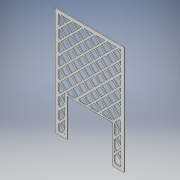
# Autodesk Inventor part: 2AM-17-07-Belly Pan
Saved by Autodesk Inventor 2017 (Build 210142000, 142)
## iProperties
Created: 2017-12-28
Part Number: 2AM-17-07-Belly Pan
Material: Generic
Document SubType Name: Modeling
Designer: anikasoojin
Density: 1 g/cm^3
Appearance: Default
Author: anikasoojin
Autodesk Inventor part; units mm, degrees
ref_plane "YZ Plane" through (0, 0, 0) normal (1, 0, 0) x (0, 1, 0)
ref_plane "XZ Plane" through (0, 0, 0) normal (0, 1, 0) x (-1, 0, 0)
ref_plane "XY Plane" through (0, 0, 0) normal (0, 0, 1) x (1, 0, 0)
sketch "Sketch1" plane through (0, 0, 0) normal (0, 0, 1) x (1, 0, 0)
  line L0 (80.4678, 8.0008) -> (613.8678, 8.0008)
  line L1 (613.8678, 8.0008) -> (613.8678, -830.1992)
  line L2 (80.4678, -830.1992) -> (80.4678, 8.0008)
  line L3 (572.8411, -17.3992) -> (588.4678, -33.0259)
  line L4 (563.8608, -26.3795) -> (588.4678, -50.9864)
  line L5 (588.4678, -17.3992) -> (572.8411, -17.3992)
  line L6 (588.4678, -33.0259) -> (588.4678, -17.3992)
  line L7 (483.0385, -17.3992) -> (518.9595, -53.3203)
  line L8 (554.8806, -17.3992) -> (518.9595, -53.3203)
  line L9 (474.0583, -26.3795) -> (509.9793, -62.3005)
  line L10 (563.8608, -26.3795) -> (527.9398, -62.3005)
  line L11 (588.4678, -76.6506) -> (588.4678, -50.9864)
  line L12 (565.3788, -99.7395) -> (588.4678, -76.6506)
  line L13 (527.9398, -62.3005) -> (565.3788, -99.7395)
  line L14 (574.3591, -108.7198) -> (588.4678, -122.8285)
  line L15 (518.9595, -71.2808) -> (556.3985, -108.7198)
  line L16 (565.3788, -117.7) -> (588.4678, -140.789)
  line L17 (574.3591, -108.7198) -> (588.4678, -94.6111)
  line L18 (588.4678, -122.8285) -> (588.4678, -94.6111)
  line L19 (554.8806, -17.3992) -> (483.0385, -17.3992)
  line L20 (465.078, -17.3992) -> (429.157, -53.3203)
  line L21 (393.236, -17.3992) -> (429.157, -53.3203)
  line L22 (384.2557, -26.3795) -> (420.1767, -62.3005)
  line L23 (474.0583, -26.3795) -> (438.1372, -62.3005)
  line L24 (438.1372, -62.3005) -> (474.0583, -98.2215)
  line L25 (509.9793, -62.3005) -> (474.0583, -98.2215)
  line L26 (429.157, -71.2808) -> (465.078, -107.2018)
  line L27 (518.9595, -71.2808) -> (483.0385, -107.2018)
  line L28 (520.4775, -144.6408) -> (556.3985, -108.7198)
  line L29 (483.0385, -107.2018) -> (520.4775, -144.6408)
  line L30 (474.0583, -116.1821) -> (511.4973, -153.6211)
  line L31 (529.4578, -153.6211) -> (565.3788, -117.7)
  line L32 (565.7758, -189.9391) -> (588.4678, -167.2472)
  line L33 (529.4578, -153.6211) -> (565.7758, -189.9391)
  line L34 (576.6156, -200.7789) -> (588.4678, -212.631)
  line L35 (520.4775, -162.6013) -> (556.7956, -198.9194)
  line L36 (567.6353, -209.7591) -> (588.4678, -230.5916)
  line L37 (576.6156, -200.7789) -> (588.4678, -188.9267)
  line L38 (588.4678, -167.2472) -> (588.4678, -140.789)
  line L39 (465.078, -107.2018) -> (429.157, -143.1228)
  line L40 (474.0583, -116.1821) -> (438.1372, -152.1031)
  line L41 (438.1372, -152.1031) -> (475.5762, -189.5421)
  line L42 (475.5762, -189.5421) -> (511.4973, -153.6211)
  line L43 (429.157, -161.0833) -> (466.596, -198.5223)
  line L44 (484.5565, -198.5223) -> (520.4775, -162.6013)
  line L45 (465.078, -17.3992) -> (393.236, -17.3992)
  line L46 (303.4334, -17.3992) -> (339.3544, -53.3203)
  line L47 (375.2754, -17.3992) -> (339.3544, -53.3203)
  line L48 (294.4531, -26.3795) -> (330.3742, -62.3005)
  line L49 (384.2557, -26.3795) -> (348.3347, -62.3005)
  line L50 (348.3347, -62.3005) -> (384.2557, -98.2215)
  line L51 (393.236, -107.2018) -> (429.157, -143.1228)
  line L52 (420.1767, -62.3005) -> (384.2557, -98.2215)
  line L53 (339.3544, -71.2808) -> (375.2754, -107.2018)
  line L54 (384.2557, -116.1821) -> (420.1767, -152.1031)
  line L55 (429.157, -71.2808) -> (393.236, -107.2018)
  line L56 (375.2754, -107.2018) -> (339.3544, -143.1228)
  line L57 (384.2557, -116.1821) -> (348.3347, -152.1031)
  line L58 (303.4334, -107.2018) -> (339.3544, -143.1228)
  line L59 (330.3742, -62.3005) -> (294.4531, -98.2215)
  line L60 (294.4531, -116.1821) -> (330.3742, -152.1031)
  line L61 (339.3544, -71.2808) -> (303.4334, -107.2018)
  line L62 (375.2754, -17.3992) -> (303.4334, -17.3992)
  line L63 (285.4729, -17.3992) -> (213.6308, -17.3992)
  line L64 (195.6703, -17.3992) -> (123.8283, -17.3992)
  line L65 (213.6308, -17.3992) -> (249.5519, -53.3203)
  line L66 (258.5321, -62.3005) -> (294.4531, -98.2215)
  line L67 (285.4729, -17.3992) -> (249.5519, -53.3203)
  line L68 (204.6506, -26.3795) -> (240.5716, -62.3005)
  line L69 (249.5519, -71.2808) -> (285.4729, -107.2018)
  line L70 (294.4531, -26.3795) -> (258.5321, -62.3005)
  line L71 (123.8283, -17.3992) -> (159.7493, -53.3203)
  line L72 (204.6506, -26.3795) -> (168.7296, -62.3005)
  line L73 (168.7296, -62.3005) -> (204.6506, -98.2215)
  line L74 (240.5716, -62.3005) -> (204.6506, -98.2215)
  line L75 (249.5519, -71.2808) -> (213.6308, -107.2018)
  line L76 (285.4729, -107.2018) -> (249.5519, -143.1228)
  line L77 (213.6308, -107.2018) -> (249.5519, -143.1228)
  line L78 (204.6506, -116.1821) -> (240.5716, -152.1031)
  line L79 (294.4531, -116.1821) -> (258.5321, -152.1031)
  line L80 (330.3742, -152.1031) -> (294.4531, -188.0241)
  line L81 (258.5321, -152.1031) -> (294.4531, -188.0241)
  line L82 (249.5519, -161.0833) -> (285.4729, -197.0044)
  line L83 (339.3544, -161.0833) -> (303.4334, -197.0044)
  line L84 (303.4334, -197.0044) -> (339.3544, -232.9254)
  line L85 (339.3544, -161.0833) -> (375.2754, -197.0044)
  line L86 (420.1767, -152.1031) -> (384.2557, -188.0241)
  line L87 (375.2754, -197.0044) -> (339.3544, -232.9254)
  line L88 (348.3347, -152.1031) -> (384.2557, -188.0241)
  line L89 (195.6703, -17.3992) -> (159.7493, -53.3203)
  line L90 (150.769, -62.3005) -> (114.848, -98.2215)
  line L91 (105.8678, -17.3992) -> (150.769, -62.3005)
  line L92 (159.7493, -71.2808) -> (195.6703, -107.2018)
  line L93 (105.8678, -89.2413) -> (114.848, -98.2215)
  line L94 (159.7493, -71.2808) -> (123.8283, -107.2018)
  line L95 (114.848, -116.1821) -> (105.8678, -125.1623)
  line L96 (105.8678, -17.3992) -> (105.8678, -89.2413)
  line L97 (114.848, -116.1821) -> (150.769, -152.1031)
  line L98 (195.6703, -107.2018) -> (159.7493, -143.1228)
  line L99 (150.769, -152.1031) -> (115.9232, -186.9489)
  line L100 (123.8283, -107.2018) -> (159.7493, -143.1228)
  line L101 (204.6506, -116.1821) -> (168.7296, -152.1031)
  line L102 (240.5716, -152.1031) -> (204.6506, -188.0241)
  line L103 (168.7296, -152.1031) -> (204.6506, -188.0241)
  line L104 (159.7493, -161.0833) -> (195.6703, -197.0044)
  line L105 (249.5519, -161.0833) -> (213.6308, -197.0044)
  line L106 (105.8678, -176.8934) -> (115.9232, -186.9489)
  line L107 (159.7493, -161.0833) -> (124.9035, -195.9292)
  line L108 (114.848, -205.9846) -> (105.8678, -214.9649)
  line L109 (588.4678, -212.631) -> (588.4678, -188.9267)
  line L110 (588.4678, -257.8438) -> (588.4678, -230.5916)
  line L111 (575.1531, -289.1189) -> (588.4678, -302.4336)
  line L112 (566.1728, -298.0992) -> (588.4678, -320.3941)
  line L113 (566.1728, -280.1387) -> (588.4678, -257.8438)
  line L114 (575.1531, -289.1189) -> (588.4678, -275.8043)
  line L115 (475.5762, -207.5026) -> (511.8943, -243.8206)
  line L116 (522.734, -254.6604) -> (557.1926, -289.1189)
  line L117 (520.8745, -234.8404) -> (556.7956, -198.9194)
  line L118 (484.5565, -198.5223) -> (520.8745, -234.8404)
  line L119 (531.7143, -245.6801) -> (566.1728, -280.1387)
  line L120 (531.7143, -245.6801) -> (567.6353, -209.7591)
  line L121 (393.236, -197.0044) -> (430.675, -234.4434)
  line L122 (430.675, -234.4434) -> (466.596, -198.5223)
  line L123 (384.2557, -205.9846) -> (421.6947, -243.4236)
  line L124 (439.6552, -243.4236) -> (475.5762, -207.5026)
  line L125 (429.157, -161.0833) -> (393.236, -197.0044)
  line L126 (384.2557, -205.9846) -> (348.3347, -241.9056)
  line L127 (294.4531, -205.9846) -> (330.3742, -241.9056)
  line L128 (475.9733, -279.7417) -> (511.8943, -243.8206)
  line L129 (439.6552, -243.4236) -> (475.9733, -279.7417)
  line L130 (430.675, -252.4039) -> (466.993, -288.7219)
  line L131 (486.813, -290.5814) -> (522.734, -254.6604)
  line L132 (105.8678, -125.1623) -> (105.8678, -176.8934)
  line L133 (195.6703, -197.0044) -> (160.8245, -231.8502)
  line L134 (150.769, -241.9056) -> (114.848, -277.8267)
  line L135 (124.9035, -195.9292) -> (160.8245, -231.8502)
  line L136 (114.848, -205.9846) -> (150.769, -241.9056)
  line L137 (204.6506, -205.9846) -> (169.8048, -240.8304)
  line L138 (285.4729, -197.0044) -> (249.5519, -232.9254)
  line L139 (213.6308, -197.0044) -> (249.5519, -232.9254)
  line L140 (294.4531, -205.9846) -> (258.5321, -241.9056)
  line L141 (204.6506, -205.9846) -> (240.5716, -241.9056)
  line L142 (258.5321, -241.9056) -> (294.4531, -277.8267)
  line L143 (330.3742, -241.9056) -> (294.4531, -277.8267)
  line L144 (249.5519, -250.8859) -> (285.4729, -286.8069)
  line L145 (339.3544, -250.8859) -> (303.4334, -286.8069)
  line L146 (339.3544, -250.8859) -> (376.7934, -288.3249)
  line L147 (385.7737, -279.3446) -> (421.6947, -243.4236)
  line L148 (348.3347, -241.9056) -> (385.7737, -279.3446)
  line L149 (394.7539, -288.3249) -> (430.675, -252.4039)
  line L150 (394.7539, -288.3249) -> (431.072, -324.643)
  line L151 (431.072, -324.643) -> (466.993, -288.7219)
  line L152 (385.7737, -297.3052) -> (422.0917, -333.6232)
  line L153 (441.9117, -335.4827) -> (477.8328, -299.5617)
  line L154 (477.8328, -299.5617) -> (512.2913, -334.0202)
  line L155 (521.2716, -325.04) -> (557.1926, -289.1189)
  line L156 (486.813, -290.5814) -> (521.2716, -325.04)
  line L157 (530.2518, -334.0202) -> (566.1728, -298.0992)
  line L158 (530.2518, -334.0202) -> (566.1728, -369.9413)
  line L159 (575.2402, -379.0087) -> (588.4678, -392.2362)
  line L160 (588.4678, -347.6463) -> (566.1728, -369.9413)
  line L161 (521.2716, -343.0005) -> (557.1926, -378.9215)
  line L162 (566.26, -387.9889) -> (588.4678, -410.1967)
  line L163 (588.4678, -365.7811) -> (575.2402, -379.0087)
  line L164 (588.4678, -302.4336) -> (588.4678, -275.8043)
  line L165 (105.8678, -268.8464) -> (114.848, -277.8267)
  line L166 (159.7493, -250.8859) -> (123.8283, -286.8069)
  line L167 (114.848, -295.7872) -> (105.8678, -304.7674)
  line L168 (105.8678, -214.9649) -> (105.8678, -268.8464)
  line L169 (114.848, -295.7872) -> (150.769, -331.7082)
  line L170 (150.769, -331.7082) -> (114.848, -367.6292)
  line L171 (123.8283, -286.8069) -> (159.7493, -322.7279)
  line L172 (240.5716, -241.9056) -> (205.7258, -276.7515)
  line L173 (195.6703, -286.8069) -> (159.7493, -322.7279)
  line L174 (169.8048, -240.8304) -> (205.7258, -276.7515)
  line L175 (159.7493, -250.8859) -> (195.6703, -286.8069)
  line L176 (249.5519, -250.8859) -> (214.706, -285.7317)
  line L177 (204.6506, -295.7872) -> (168.7296, -331.7082)
  line L178 (285.4729, -286.8069) -> (250.6271, -321.6527)
  line L179 (214.706, -285.7317) -> (250.6271, -321.6527)
  line L180 (204.6506, -295.7872) -> (240.5716, -331.7082)
  line L181 (294.4531, -295.7872) -> (259.6073, -330.633)
  line L182 (303.4334, -286.8069) -> (340.8724, -324.2459)
  line L183 (340.8724, -324.2459) -> (376.7934, -288.3249)
  line L184 (294.4531, -295.7872) -> (331.8921, -333.2262)
  line L185 (349.8527, -333.2262) -> (385.7737, -297.3052)
  line L186 (588.4678, -347.6463) -> (588.4678, -320.3941)
  line L187 (588.4678, -392.2362) -> (588.4678, -365.7811)
  line L188 (441.9117, -335.4827) -> (476.3703, -369.9413)
  line L189 (476.3703, -369.9413) -> (512.2913, -334.0202)
  line L190 (432.9315, -344.463) -> (467.39, -378.9215)
  line L191 (485.3505, -378.9215) -> (521.2716, -343.0005)
  line L192 (349.8527, -333.2262) -> (386.1707, -369.5442)
  line L193 (386.1707, -369.5442) -> (422.0917, -333.6232)
  line L194 (340.8724, -342.2064) -> (377.1904, -378.5245)
  line L195 (397.0104, -380.384) -> (432.9315, -344.463)
  line L196 (259.6073, -330.633) -> (297.0463, -368.072)
  line L197 (297.0463, -368.072) -> (331.8921, -333.2262)
  line L198 (249.5519, -340.6885) -> (286.9909, -378.1275)
  line L199 (306.0266, -377.0523) -> (340.8724, -342.2064)
  line L200 (168.7296, -331.7082) -> (204.6506, -367.6292)
  line L201 (240.5716, -331.7082) -> (204.6506, -367.6292)
  line L202 (159.7493, -340.6885) -> (195.6703, -376.6095)
  line L203 (249.5519, -340.6885) -> (213.6308, -376.6095)
  line L204 (397.0104, -380.384) -> (431.469, -414.8425)
  line L205 (431.469, -414.8425) -> (467.39, -378.9215)
  line L206 (388.0302, -389.3642) -> (422.4888, -423.8228)
  line L207 (440.4493, -423.8228) -> (476.3703, -387.9018)
  line L208 (476.3703, -387.9018) -> (512.2913, -423.8228)
  line L209 (557.1926, -378.9215) -> (521.2716, -414.8425)
  line L210 (485.3505, -378.9215) -> (521.2716, -414.8425)
  line L211 (530.339, -423.9099) -> (577.7767, -471.3477)
  line L212 (566.26, -387.9889) -> (530.339, -423.9099)
  line L213 (105.8678, -358.649) -> (114.848, -367.6292)
  line L214 (105.8678, -304.7674) -> (105.8678, -358.649)
  line L215 (159.7493, -340.6885) -> (123.8283, -376.6095)
  line L216 (114.848, -385.5897) -> (105.8678, -394.57)
  line L217 (123.8283, -376.6095) -> (159.7493, -412.5305)
  line L218 (195.6703, -376.6095) -> (159.7493, -412.5305)
  line L219 (150.769, -421.5108) -> (114.848, -457.4318)
  line L220 (114.848, -385.5897) -> (150.769, -421.5108)
  line L221 (204.6506, -385.5897) -> (168.7296, -421.5108)
  line L222 (251.0698, -414.0485) -> (286.9909, -378.1275)
  line L223 (213.6308, -376.6095) -> (251.0698, -414.0485)
  line L224 (204.6506, -385.5897) -> (242.0896, -423.0287)
  line L225 (260.0501, -423.0287) -> (295.9711, -387.1077)
  line L226 (342.3446, -413.3703) -> (377.1904, -378.5245)
  line L227 (306.0266, -377.0523) -> (342.3446, -413.3703)
  line L228 (295.9711, -387.1077) -> (332.2892, -423.4258)
  line L229 (353.1844, -424.21) -> (388.0302, -389.3642)
  line L230 (168.7296, -421.5108) -> (206.1686, -458.9498)
  line L231 (206.1686, -458.9498) -> (242.0896, -423.0287)
  line L232 (159.7493, -430.491) -> (197.1883, -467.93)
  line L233 (215.1488, -467.93) -> (251.0698, -432.009)
  line L234 (105.8678, -448.4515) -> (114.848, -457.4318)
  line L235 (159.7493, -430.491) -> (123.8283, -466.412)
  line L236 (114.848, -475.3923) -> (105.8678, -484.3726)
  line L237 (105.8678, -394.57) -> (105.8678, -448.4515)
  line L238 (114.848, -475.3923) -> (152.287, -512.8313)
  line L239 (116.366, -548.7523) -> (152.287, -512.8313)
  line L240 (161.2673, -503.8511) -> (197.1883, -467.93)
  line L241 (123.8283, -466.412) -> (161.2673, -503.8511)
  line L242 (170.2475, -512.8313) -> (206.1686, -476.9103)
  line L243 (353.1844, -424.21) -> (387.6429, -458.6686)
  line L244 (387.6429, -458.6686) -> (422.4888, -423.8228)
  line L245 (343.1289, -434.2655) -> (377.5875, -468.7241)
  line L246 (396.6232, -467.6489) -> (431.469, -432.803)
  line L247 (440.4493, -423.8228) -> (476.3703, -459.7438)
  line L248 (512.2913, -423.8228) -> (476.3703, -459.7438)
  line L249 (431.469, -432.803) -> (467.39, -468.7241)
  line L250 (521.3587, -432.8902) -> (485.4377, -468.8112)
  line L251 (341.6664, -504.6451) -> (377.5875, -468.7241)
  line L252 (350.6467, -513.6254) -> (386.5677, -477.7043)
  line L253 (350.6467, -513.6254) -> (362.4206, -525.3992)
  line L254 (341.6664, -522.6056) -> (344.4601, -525.3992)
  line L255 (215.1488, -467.93) -> (251.4669, -504.2481)
  line L256 (206.1686, -476.9103) -> (242.4866, -513.2283)
  line L257 (262.3066, -515.0878) -> (272.618, -525.3992)
  line L258 (320.9123, -525.3992) -> (332.6862, -513.6254)
  line L259 (338.8728, -525.3992) -> (341.6664, -522.6056)
  line L260 (260.0501, -423.0287) -> (296.3681, -459.3468)
  line L261 (307.2079, -470.1865) -> (341.6664, -504.6451)
  line L262 (251.4669, -504.2481) -> (287.3879, -468.327)
  line L263 (296.3681, -459.3468) -> (332.2892, -423.4258)
  line L264 (251.0698, -432.009) -> (287.3879, -468.327)
  line L265 (298.2276, -479.1668) -> (332.6862, -513.6254)
  line L266 (262.3066, -515.0878) -> (298.2276, -479.1668)
  line L267 (307.2079, -470.1865) -> (343.1289, -434.2655)
  line L268 (521.3587, -432.8902) -> (568.7965, -480.328)
  line L269 (579.4875, -491.019) -> (588.4678, -499.9992)
  line L270 (588.4678, -460.6567) -> (577.7767, -471.3477)
  line L271 (588.4678, -460.6567) -> (588.4678, -410.1967)
  line L272 (588.4678, -571.8413) -> (588.4678, -499.9992)
  line L273 (476.4574, -477.7915) -> (523.8952, -525.2292)
  line L274 (537.6678, -539.0018) -> (579.8256, -581.1596)
  line L275 (568.7965, -480.328) -> (532.8755, -516.249)
  line L276 (485.4377, -468.8112) -> (532.8755, -516.249)
  line L277 (543.5665, -526.94) -> (588.4678, -571.8413)
  line L278 (543.5665, -526.94) -> (579.4875, -491.019)
  line L279 (386.5677, -477.7043) -> (422.4888, -513.6254)
  line L280 (467.39, -468.7241) -> (432.5442, -503.5699)
  line L281 (422.4888, -513.6254) -> (410.7149, -525.3992)
  line L282 (396.6232, -467.6489) -> (432.5442, -503.5699)
  line L283 (476.4574, -477.7915) -> (441.6116, -512.6373)
  line L284 (431.5561, -522.6927) -> (428.8497, -525.3992)
  line L285 (441.6116, -512.6373) -> (454.3736, -525.3992)
  line L286 (523.8952, -525.2292) -> (523.7252, -525.3992)
  line L287 (431.5561, -522.6927) -> (434.2626, -525.3992)
  line L288 (537.6678, -608.6934) -> (546.2915, -617.3172)
  line L289 (554.9337, -625.9594) -> (588.4678, -659.4934)
  line L290 (546.2915, -617.3172) -> (579.8256, -581.1596)
  line L291 (545.2568, -636.3934) -> (588.4678, -679.6044)
  line L292 (554.9337, -625.9594) -> (588.4678, -589.8018)
  line L293 (588.4678, -659.4934) -> (588.4678, -589.8018)
  line L294 (537.6678, -644.5761) -> (545.2568, -636.3934)
  line L295 (537.6678, -700.6464) -> (553.899, -716.8776)
  line L296 (562.414, -725.3926) -> (588.4678, -751.4464)
  line L297 (588.4678, -679.6044) -> (553.899, -716.8776)
  line L298 (537.6678, -718.6069) -> (545.2568, -726.1959)
  line L299 (553.7718, -734.7109) -> (588.4678, -769.4069)
  line L300 (588.4678, -697.3005) -> (562.414, -725.3926)
  line L301 (588.4678, -804.7992) -> (588.4678, -769.4069)
  line L302 (588.4678, -751.4464) -> (588.4678, -697.3005)
  line L303 (552.018, -804.7992) -> (588.4678, -804.7992)
  line L304 (553.7718, -734.7109) -> (537.6678, -752.0749)
  line L305 (545.2568, -726.1959) -> (537.6678, -734.3787)
  line L306 (537.6678, -790.449) -> (552.018, -804.7992)
  line L307 (114.8484, -640.8666) -> (150.7707, -604.9442)
  line L308 (114.7696, -568.3092) -> (150.7707, -604.9442)
  line L309 (105.8678, -631.7279) -> (114.8484, -640.8666)
  line L310 (105.8678, -671.5267) -> (116.6129, -660.7815)
  line L311 (125.5935, -651.8009) -> (156.6678, -620.7267)
  line L312 (125.5935, -651.8009) -> (156.6678, -683.4223)
  line L313 (114.8484, -731.4632) -> (150.7707, -695.5408)
  line L314 (116.6129, -660.7815) -> (150.7707, -695.5408)
  line L315 (105.8678, -722.3245) -> (114.8484, -731.4632)
  line L316 (105.8678, -758.4043) -> (114.7696, -749.5024)
  line L317 (123.7502, -740.5218) -> (156.6678, -707.6043)
  line L318 (105.8678, -671.5267) -> (105.8678, -722.3245)
  line L319 (105.8678, -758.4043) -> (105.8678, -804.7992)
  line L320 (123.7502, -740.5218) -> (156.6678, -774.0189)
  line L321 (150.3772, -785.7369) -> (131.3149, -804.7992)
  line L322 (114.7696, -749.5024) -> (150.3772, -785.7369)
  line L323 (156.6678, -797.5811) -> (149.4497, -804.7992)
  line L324 (105.8678, -804.7992) -> (131.3149, -804.7992)
  line L325 (149.4497, -804.7992) -> (156.6678, -804.7992)
  line L326 (230.3157, -525.3992) -> (242.4866, -513.2283)
  line L327 (170.2475, -512.8313) -> (182.8155, -525.3992)
  line L328 (105.8678, -538.2541) -> (116.366, -548.7523)
  line L329 (125.3463, -557.7326) -> (156.6678, -589.0541)
  line L330 (105.8678, -577.2111) -> (114.7696, -568.3092)
  line L331 (105.8678, -484.3726) -> (105.8678, -538.2541)
  line L332 (105.8678, -577.2111) -> (105.8678, -631.7279)
  line L333 (525.7456, -804.7992) -> (525.7456, -538.2541)
  line L334 (525.7456, -538.2541) -> (172.504, -538.2541)
  line L335 (172.504, -538.2541) -> (172.504, -804.7992)
  line L336 (523.7252, -525.3992) -> (454.3736, -525.3992)
  line L337 (434.2626, -525.3992) -> (428.8497, -525.3992)
  line L338 (537.6678, -608.6934) -> (537.6678, -539.0018)
  line L339 (537.6678, -700.6464) -> (537.6678, -644.5761)
  line L340 (537.6678, -790.449) -> (537.6678, -752.0749)
  line L341 (537.6678, -734.3787) -> (537.6678, -718.6069)
  line L342 (410.7149, -525.3992) -> (362.4206, -525.3992)
  line L343 (344.4601, -525.3992) -> (338.8728, -525.3992)
  line L344 (320.9123, -525.3992) -> (272.618, -525.3992)
  line L345 (230.3157, -525.3992) -> (182.8155, -525.3992)
  line L346 (156.6678, -526.4111) -> (156.6678, -589.0541)
  line L347 (156.6678, -620.7267) -> (156.6678, -683.4223)
  line L348 (156.6678, -707.6043) -> (156.6678, -774.0189)
  line L349 (156.6678, -797.5811) -> (156.6678, -804.7992)
  line L350 (125.3463, -557.7326) -> (156.6678, -526.4111)
  line L351 (525.7456, -804.7992) -> (525.7456, -830.1992)
  line L352 (172.504, -804.7992) -> (172.504, -830.1992)
  line L353 (613.8678, -830.1992) -> (525.7456, -830.1992)
  line L354 (172.504, -830.1992) -> (80.4678, -830.1992)
  line L355 (156.6678, -830.1992) -> (172.504, -830.1992)
  line L356 (525.7456, -830.1992) -> (537.6678, -830.1992)
  point P0 (0, 0)
  point P1 (397.86, -538.2541)
  point P2 (308.0575, -538.2541)
  point P3 (510.8703, -538.2541)
  point P4 (525.7456, -596.7713)
  point P5 (492.241, -475.6145)
  point P6 (525.7456, -688.7243)
  point P7 (501.7467, -525.3992)
  point P8 (525.7456, -764.9297)
  point P9 (525.7456, -796.4874)
  point P10 (172.504, -673.8075)
  point P11 (172.504, -699.5374)
  point P12 (172.504, -717.6568)
  point P13 (177.7098, -538.2541)
  point P14 (217.4608, -538.2541)
  dimension "d0" = 533.4
  dimension "d1" = 838.2
  dimension "d4" = 12.7
  constraints: 1574 parallel, 714 end point, 321 perpendicular, 15 point on line, 3 horizontal, 1 vertical
  measures "d0" distance of L0.start L0.end
  measures "d1" distance of L0.end L1.end
  measures "d4" distance between parallel lines of L3 L4
extrude "Extrusion2" add sketch "Sketch1" along normal blind 6.35
body "Solid2"
